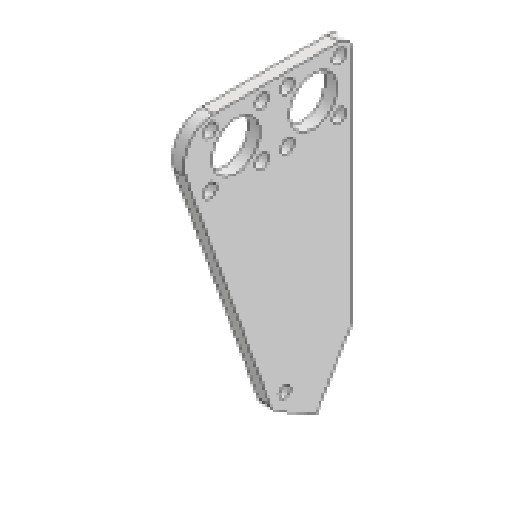
# Autodesk Inventor part: verticalSlidesPlate
Saved by Autodesk Inventor 2023 (Build 270158000, 158)
## iProperties
Created: 2022-10-26
Part Number: verticalSlidesPlate
Material: Generic
Document SubType Name: Modeling
Designer: deli
Density: 1 g/cm^3
Appearance: Default
Author: deli
Autodesk Inventor part; units mm, degrees
ref_plane "YZ Plane" through (0, 0, 0) normal (1, 0, 0) x (0, 1, 0)
ref_plane "XZ Plane" through (0, 0, 0) normal (0, 1, 0) x (-1, 0, 0)
ref_plane "XY Plane" through (0, 0, 0) normal (0, 0, 1) x (1, 0, 0)
sketch "Sketch1" plane through (0, 0, 0) normal (1, 0, 0) x (0, 1, 0)
  line L0 (483.6699, -478.5728) -> (473.1693, -495.5945) construction
  line L1 (473.1693, -495.5945) -> (217.8443, -338.0853) construction
  line L2 (217.8443, -338.0853) -> (228.3449, -321.0636) construction
  line L3 (228.3449, -321.0636) -> (483.6699, -478.5728) construction
  line L4 (228.3449, -321.0636) -> (-358.9027, 41.2074) construction
  line L5 (-358.9027, 41.2074) -> (-369.4033, 24.1858) construction
  line L6 (-369.4033, 24.1858) -> (217.8443, -338.0853) construction
  line L7 (-499.9626, 206.2365) -> (-499.9626, -867.2165) construction
  line L8 (-358.9027, 41.2074) -> (-362.7325, 43.5701) construction
  line L9 (-362.7325, 43.5701) -> (-373.2331, 26.5484) construction
  line L10 (-373.2331, 26.5484) -> (-369.4033, 24.1858) construction
  line L11 (-379.9626, 138.1186) -> (-379.9626, -322.1895) construction
  line L12 (-362.7325, 43.5701) -> (-371.6689, 49.0829) construction
  line L13 (-371.6689, 49.0829) -> (-369.9626, 51.8489) construction
  circle A0 centre (465.6533, -479.2082) radius 1.6
  circle A1 centre (350.7571, -408.3291) radius 1.6 construction
  circle A2 centre (235.8608, -337.4499) radius 1.6 construction
  line L14 (350.9374, -635.582) -> (-499.9626, -635.582) construction
  line L15 (350.9374, -635.582) -> (350.9374, -660.982) construction
  line L16 (350.9374, -660.982) -> (-499.9626, -660.982) construction
  circle A3 centre (-53.3626, -143.4606) radius 4.25 construction
  line L17 (-451.9626, 107.1246) -> (-451.9626, -344.4416) construction
  line L18 (483.6699, -478.5728) -> (532.1817, -508.4995) construction
  circle A4 centre (534.413, -504.8824) radius 4.25 construction
  line L19 (386.8939, -540.5479) -> (363.6374, -540.5479) construction
  line L20 (363.6374, -540.5479) -> (363.6374, -642.1479) construction
  line L21 (363.6374, -642.1479) -> (386.8939, -642.1479) construction
  line L22 (386.8939, -550.0729) -> (490.6374, -565.9479) construction
  line L23 (490.6374, -565.9479) -> (490.6374, -616.7479) construction
  line L24 (490.6374, -616.7479) -> (386.8939, -632.6229) construction
  line L25 (386.8939, -642.1479) -> (386.8939, -632.6229) construction
  line L26 (386.8939, -550.0729) -> (386.8939, -540.5479) construction
  line L27 (455.9486, -487.3211) -> (462.249, -477.1081)
  arc A5 (464.3226, -475.436) -> (462.249, -477.1081) centre (465.6533, -479.2082) ccw
  line L28 (455.9486, -487.3211) -> (472.1192, -497.2966)
  circle A6 centre (528.376, -487.0096) radius 6.35
  circle A7 centre (535.2908, -493.9244) radius 1.8288
  circle A8 centre (521.4612, -493.9244) radius 1.8288
  circle A9 centre (521.4612, -480.0948) radius 1.8288
  circle A10 centre (535.2908, -480.0948) radius 1.8288
  circle A11 centre (528.376, -487.0096) radius 7.9502 construction
  line L29 (535.2908, -480.0948) -> (535.2908, -493.9244) construction
  line L30 (535.2908, -493.9244) -> (521.4612, -493.9244) construction
  circle A12 centre (528.376, -466.4356) radius 6.35
  circle A13 centre (535.2908, -473.3504) radius 1.8288
  circle A14 centre (521.4612, -473.3504) radius 1.8288
  circle A15 centre (521.4612, -459.5208) radius 1.8288
  circle A16 centre (535.2908, -459.5208) radius 1.8288
  circle A17 centre (528.376, -466.4356) radius 7.9502 construction
  line L31 (535.2908, -459.5208) -> (535.2908, -473.3504) construction
  line L32 (535.2908, -473.3504) -> (521.4612, -473.3504) construction
  line L33 (472.1192, -497.2966) -> (535.2908, -497.2966)
  line L34 (538.663, -493.9244) -> (538.663, -460.5163)
  line L35 (528.0016, -452.972) -> (464.3226, -475.436)
  arc A18 (538.663, -460.5163) -> (528.0016, -452.972) centre (530.663, -460.5163) ccw
  arc A19 (535.2908, -497.2966) -> (538.663, -493.9244) centre (535.2908, -493.9244) ccw
  point P0 (0, 0)
  point P1 (-370.8157, 50.4659)
  dimension "d24" = 8.5
  dimension "d0" = 20
  dimension "d1" = 300
  dimension "d2" = 690
  dimension "d3" = 4.5
  dimension "d4" = 120
  dimension "d5" = 10.5
  dimension "d6" = 3.25
  dimension "d7" = 10
  dimension "d8" = 3.2
  dimension "d9" = 10
  dimension "d10" = 10
  dimension "d11" = 10
  dimension "d12" = 15
  dimension "d13" = 135
  dimension "d14" = 135
  dimension "d15" = 25.4
  dimension "d16" = 850.9
  dimension "d17" = 8.5
  dimension "d18" = 3.25
  dimension "d19" = 372
  dimension "d21" = 48
  dimension "d22" = 398.6
  dimension "d23" = 57
  dimension "d26" = 101.6
  dimension "d27" = 50.8
  dimension "d28" = 8.7
  dimension "d29" = 8.7
  dimension "d30" = 127
  dimension "d31" = 82.55
  dimension "d32" = 904.3756
  dimension "d33" = 12.7
  dimension "d34" = 48.0256
  dimension "d36" = 8
  dimension "d37" = 2
  dimension "d38" = 12.7
  dimension "d39" = 3.6576
  dimension "d40" = 19.558
  dimension "d41" = 19.558
  dimension "d42" = 6.037
  dimension "d43" = 12.7
  dimension "d44" = 3.6576
  dimension "d45" = 19.558
  dimension "d46" = 19.558
  dimension "d47" = 6.037
  dimension "d48" = 20.574
  dimension "d49" = 10.287
  dimension "d50" = 4
  dimension "d51" = 10.287
  dimension "d52" = 8
  constraints: 72 end point, 19 centre point, 15 perpendicular, 13 tangent, 8 equal radius, 6 point on circle, 6 vertical, 5 coincident, 5 parallel, 4 collinear, 4 point on line, 3 equal length, 3 horizontal, 1 concentric, 1 midpoint, 4 other
  measures "d0" distance of L0.start L0.end
  measures "d1" distance of L2.end L0.start
  measures "d2" distance of L2.end L4.end
  measures "d3" distance of L4.end L8.end
  measures "d4" distance between parallel lines of L11 L7
  measures "d5" distance of L8.end L12.end
  measures "d6" distance of L12.end L13.end
  measures "d7" distance from line of L11 L13.end
  measures "d8" diameter of A0
  measures "d9" distance from line of L3 A0.centre
  measures "d10" distance from line of L3 A1.centre
  measures "d11" distance from line of L3 A2.centre
  measures "d12" distance from line of L0 A0.centre
  measures "d13" distance of A0.centre A1.centre
  measures "d14" distance of A2.centre A1.centre
  measures "d15" distance of L14.start L15.end
  measures "d16" distance of L14.start L14.end
  measures "d17" diameter of A3
  measures "d18" distance from line of L4 A3.centre
  measures "d19" distance of point (-370.816, 50.466) A3.centre
  measures "d21" distance between parallel lines of L17 L7
  measures "d22" distance from line of L17 A3.centre
  measures "d23" distance of L0.start L18.end
  measures "d26" distance of L20.end L19.end
  measures "d27" distance of L22.end L23.end
  measures "d28" angle of L21 L24
  measures "d29" angle of L22 L19
  measures "d30" distance between parallel lines of L20 L23
  measures "d31" distance of L24.end L22.start
  measures "d32" horizontal distance of point (534.413, -504.882) L13.end
  measures "d33" distance between parallel lines of L20 L15
  measures "d36" diameter of A5
  measures "d37" distance between parallel lines of L28 L1
  measures "d38" diameter of A6
  measures "d39" diameter of A7
  measures "d40" distance of L30.end L29.start
  measures "d41" distance of A7.centre A9.centre
  measures "d42" horizontal distance of A6.centre point (534.413, -504.882)
  measures "d43" diameter of A12
  measures "d44" diameter of A13
  measures "d45" distance of L32.end L31.start
  measures "d46" distance of A13.centre A15.centre
  measures "d47" horizontal distance of point (534.413, -504.882) A12.centre
  measures "d48" distance of A6.centre A12.centre
  measures "d49" distance from line of L33 A6.centre
  measures "d50" distance from line of A15.centre L35
  measures "d51" distance from line of L34 A11.centre
  measures "d52" radius of A18
extrude "Extrusion1" add sketch "Sketch1" along normal blind 3.175
sketch "Sketch2" plane through (0, 0, 0) normal (-1, 0, 0) x (0, 0, 1)
  line L0 (-497.2966, 472.1192) -> (-497.2966, 535.2908) projected
  line L1 (-497.2966, 472.1192) -> (-495.5945, 473.1693)
  line L2 (-495.5945, 473.1693) -> (-485.6189, 456.9987)
  line L3 (-477.1081, 462.249) -> (-487.3211, 455.9486) projected
  line L4 (-487.3211, 455.9486) -> (-497.2966, 472.1192) projected
  point P0 (0, 0)
  dimension "d55" = 2
  constraints: 4 end point, 2 perpendicular, 1 point on line
  measures "d55" distance between parallel lines of L2 L4
extrude "Extrusion2" add sketch "Sketch2" along normal blind 3.175
equation "\"d9\" = 0.5 * d0"
equation "\"d10\" = d9"
equation "\"d11\" = d10"
equation "\"d13\" = -d12 + 0.5 * d1"
equation "\"d14\" = d13"
equation "\"d18\" = d6"
equation "\"d29\" = d28"
body "Solid1"
